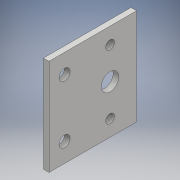
# Autodesk Inventor part: BEARING BRACKET MOUNT
Saved by Autodesk Inventor 2018 (Build 220112000, 112)
## iProperties
Created: 2018-10-15
Part Number: BEARING BRACKET MOUNT
Material: Generic
Document SubType Name: Modeling
Designer: Matthew Morey
Density: 1 g/cm^3
Appearance: Default
Author: Matthew Morey
Autodesk Inventor part; units mm, degrees
ref_plane "YZ Plane" through (0, 0, 0) normal (1, 0, 0) x (0, 1, 0)
ref_plane "XZ Plane" through (0, 0, 0) normal (0, 1, 0) x (-1, 0, 0)
ref_plane "XY Plane" through (0, 0, 0) normal (0, 0, 1) x (1, 0, 0)
sketch "Sketch1" plane through (0, 0, 0) normal (1, 0, 0) x (0, 1, 0)
  line L0 (25, 27.5) -> (-25, 27.5)
  line L1 (-25, 27.5) -> (-25, -27.5)
  line L2 (-25, -27.5) -> (25, -27.5)
  line L3 (25, -27.5) -> (25, 27.5)
  point P0 (0, 0)
  dimension "d0" = 55
  dimension "d1" = 50
  dimension "d2" = 27.5
  dimension "d3" = 25
  constraints: 8 end point, 2 parallel, 1 horizontal, 1 perpendicular
  measures "d0" distance of L2.end L0.start
  measures "d1" distance of L1.end L2.end
  measures "d2" distance from line of point (0, 0) L2
  measures "d3" distance from line of point (0, 0) L3
extrude "Extrusion1" add sketch "Sketch1" along normal blind 3.175
sketch "Sketch2" plane through (3.175, 0, 0) normal (1, 0, 0) x (0, 0, -1)
  circle A0 centre (-18.25, 9.85) radius 2.5
  circle A1 centre (18.25, 9.85) radius 2.5
  circle A2 centre (-16.5, -16.15) radius 3.175
  circle A3 centre (16.5, -16.15) radius 3.175
  line L0 (27.5, -25) -> (27.5, 25) projected
  line L1 (-27.5, 25) -> (-27.5, -25) projected
  line L2 (-27.5, -25) -> (27.5, -25) projected
  point P0 (0, 0)
  dimension "d6" = 6.35
  dimension "d8" = 11
  dimension "d9" = 11
  dimension "d10" = 6.35
  dimension "d11" = 5
  dimension "d12" = 5
  dimension "d13" = 36.5
  dimension "d14" = 9.25
  dimension "d16" = 8.85
  dimension "d17" = 8.85
  dimension "d22" = 34.85
  dimension "d23" = 34.85
  dimension "d24" = 9.25
  constraints: 4 centre point
  measures "d6" diameter of A2
  measures "d8" distance from line of L0 A3.centre
  measures "d9" distance from line of L1 A2.centre
  measures "d10" diameter of A3
  measures "d11" diameter of A0
  measures "d12" diameter of A1
  measures "d13" distance of A1.centre A0.centre
  measures "d14" distance from line of L1 A0.centre
  measures "d16" distance from line of A2.centre L2
  measures "d17" distance from line of L2 A3.centre
  measures "d22" distance from line of L2 A1.centre
  measures "d23" distance from line of L2 A0.centre
  measures "d24" distance from line of L0 A1.centre
extrude "Extrusion2" cut sketch "Sketch2" against normal through all
sketch "Sketch3" plane through (3.175, 0, 0) normal (1, 0, 0) x (0, 0, -1)
  circle A0 centre (0, 9.838) radius 5
  line L0 (27.5, -25) -> (27.5, 25) projected
  line L1 (27.5, 25) -> (-27.5, 25) projected
  point P0 (0, 0)
  dimension "d25" = 10
  dimension "d26" = 27.5
  dimension "d27" = 15.162
  constraints: 1 centre point
  measures "d25" diameter of A0
  measures "d26" distance from line of L0 A0.centre
  measures "d27" distance from line of L1 A0.centre
extrude "Extrusion3" cut sketch "Sketch3" against normal through all
body "Solid1"
